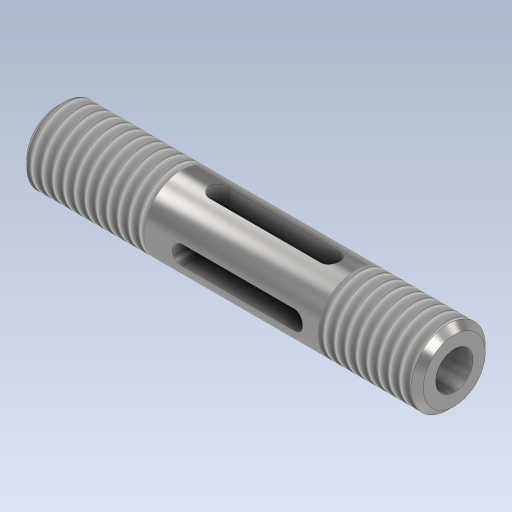
# Autodesk Inventor part: Pump-Motor-CW-Rotation:S Barrel
Saved by Autodesk Inventor 2024.2 (Build 282272000, 272)
## iProperties
Created: 2025-06-16
Material: Stainless Steel
Document SubType Name: Modeling
Density: 8 g/cm^3
Appearance: Semi-Polished
Designer: cw
Author: cw
Autodesk Inventor part; units mm, degrees
ref_plane "YZ Plane" through (0, 0, 0) normal (1, 0, 0) x (0, 1, 0)
ref_plane "XZ Plane" through (0, 0, 0) normal (0, 1, 0) x (-1, 0, 0)
ref_plane "XY Plane" through (0, 0, 0) normal (0, 0, 1) x (1, 0, 0)
sketch "Sketch1" plane through (0, 0, 0) normal (1, 0, 0) x (0, 1, 0)
  circle A0 centre (0, 0) radius 6
  circle A1 centre (0, 0) radius 3
  dimension "d0" = 12
  dimension "d7" = 6
  constraints: 2 centre point, 2 coincident
  measures "d0" diameter of A0
  measures "d7" diameter of A1
extrude "Extrusion1" add sketch "Sketch1" along normal mid plane 64
thread "Thread1" size "M12x1.75" class "6g" standard "ISO Metric profile" length 20
thread "Thread2" size "M12x1.75" class "6g" standard "ISO Metric profile" length 16
sketch "Sketch2" plane through (0, 0, 0) normal (0, 0, 1) x (1, 0, 0)
  line L0 (-6, 0) -> (12, 0) construction
  line L1 (-6, -1.5) -> (12, -1.5)
  line L2 (12, 1.5) -> (-6, 1.5)
  arc A0 (-6, 1.5) -> (-6, -1.5) centre (-6, 0) ccw
  arc A1 (12, -1.5) -> (12, 1.5) centre (12, 0) ccw
  line L3 (32, -6) -> (32, 6) projected
  point P0 (0, 0)
  point P1 (3, 0)
  dimension "d8" = 18
  dimension "d10" = 3
  dimension "d11" = 20
  constraints: 8 end point, 4 point on circle, 4 tangent, 2 centre point, 1 horizontal, 1 midpoint, 1 parallel, 1 point on line
  measures "d8" distance of L0.start L0.end
  measures "d10" distance between parallel lines of L1 L2
  measures "d11" distance from line of L3 L0.end
extrude "Extrusion2" cut sketch "Sketch2" along normal through all both and the other way through all
pattern_circular "Circular Pattern1" count 2 over 90 about axis through (0, 0, 0) along (1, 0, 0) of "Extrusion2"
chamfer "Chamfer1" distance 1 angle 45 2 edges at (-32, -6, 0) (32, -6, 0)
body "Solid1"
